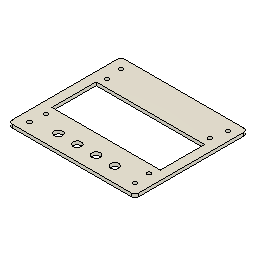
FCM Faceplate (Autodesk Fusion 360 design; units mm, degrees)
Autodesk Fusion 360 part; units mm, degrees
sketch "Sketch1" plane through (0, 0, 0) normal (0, 1, 0) x (1, 0, 0)
  arc A0 (111.125, 0) -> (114.3, 3.175) centre (111.125, 3.175) ccw
  line L0 (0, 0) -> (114.3, 0)
  line L1 (114.3, 0) -> (114.3, 101.6)
  arc A1 (3.175, 101.6) -> (0, 98.425) centre (3.175, 98.425) ccw
  arc A2 (0, 3.175) -> (3.175, 0) centre (3.175, 3.175) ccw
  circle A3 centre (25.4, 50.8) radius 3.175
  circle A4 centre (88.9, 50.8) radius 3.175
  line L2 (0, 101.6) -> (0, 0)
  line L3 (114.3, 101.6) -> (0, 101.6)
  arc A5 (114.3, 98.425) -> (111.125, 101.6) centre (111.125, 98.425) ccw
  line L4 (8.1496, 70.993) -> (8.1496, 30.988)
  line L5 (106.1504, 70.993) -> (8.1496, 70.993)
  line L6 (8.1496, 30.988) -> (106.1504, 30.988)
  line L7 (106.1504, 80.6374) -> (8.1496, 80.6374)
  line L8 (8.1496, 20.6375) -> (106.1504, 20.6375)
  line L9 (106.1504, 20.6375) -> (106.1504, 80.6374)
  line L10 (8.1496, 80.6374) -> (8.1496, 20.6375)
  line L11 (106.1504, 30.988) -> (106.1504, 70.993)
  circle A6 centre (65.3796, 13.716) radius 3.683
  circle A7 centre (48.4378, 13.716) radius 3.683
  circle A8 centre (82.3214, 13.716) radius 3.683
  circle A9 centre (31.4198, 13.716) radius 3.683
  circle A10 centre (103.6498, 23.241) radius 1.778
  circle A11 centre (10.6528, 23.241) radius 1.778
  circle A12 centre (10.6528, 78.2422) radius 1.778
  circle A13 centre (103.6498, 78.2422) radius 1.778
  circle A14 centre (9.525, 92.075) radius 1.778
  circle A15 centre (9.525, 9.525) radius 1.778
  circle A16 centre (104.775, 9.525) radius 1.778
  circle A17 centre (106.045, 92.075) radius 1.778
extrude "Extrude1" add sketch "Sketch1" along normal blind 2.9972 contours A0 L0 L1 A1 A2 L2 L3 A5 | L5 L7 L9 L10 | L6 L8 L9 L10
